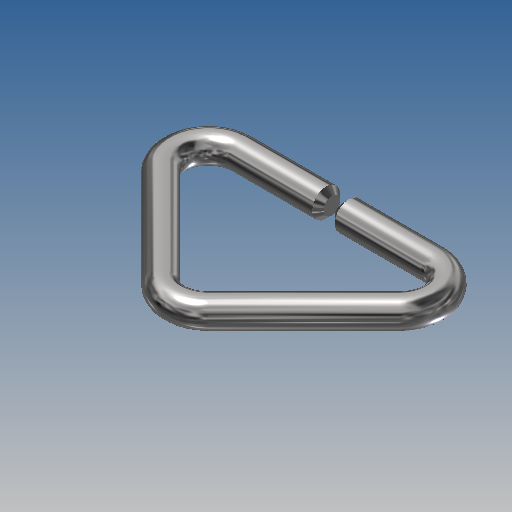
# Autodesk Inventor part: DD_KVD_002_12
Saved by Autodesk Inventor 2017.3 (Build 213256000, 256)
## iProperties
Created: 2023-12-14
Part Number: DD_KVD_002_12
Material: Nerezová ocel
Document SubType Name: Modeling
Designer: Darena
Manufacturer: Standard
Standards Organization: Custom
Density: 8 g/cm^3
Appearance: Pololeštěná
Author: Darena
Autodesk Inventor part; units mm, degrees
ref_plane "YZ Plane" through (0, 0, 0) normal (1, 0, 0) x (0, 1, 0)
ref_plane "XZ Plane" through (0, 0, 0) normal (0, 1, 0) x (-1, 0, 0)
ref_plane "XY Plane" through (0, 0, 0) normal (0, 0, 1) x (1, 0, 0)
sketch "Náčrt2" plane through (0, 0, 0) normal (0, 1, 0) x (-1, 0, 0)
  line L0 (-15, 3.4854) -> (17, 3.4854) construction
  line L1 (17, 3.4854) -> (17, 9.4853) construction
  line L2 (17, 9.4853) -> (-15, 9.4853) construction
  line L3 (20.5, 23.4853) -> (39.8276, 23.4853) construction
  line L4 (20.5, 23.4853) -> (20.5, 35.0341) construction
  line L5 (4.2426, 27.2426) -> (21.2426, 10.2426)
  line L6 (17, 0) -> (-17, 0)
  line L7 (-4.2426, 27.2426) -> (-21.2426, 10.2426)
  line L8 (0, 9.4853) -> (0, 31.4853) construction
  arc A0 (4.2426, 27.2426) -> (-4.2426, 27.2426) centre (0, 23) ccw
  arc A1 (17, 0) -> (21.2426, 10.2426) centre (17, 6) ccw
  arc A2 (-21.2426, 10.2426) -> (-17, 0) centre (-17, 6) ccw
  line L9 (19.1213, 8.1213) -> (2.1213, 25.1213) construction
  arc A3 (2.1213, 25.1213) -> (-2.1213, 25.1213) centre (0, 23) ccw construction
  line L10 (-2.1213, 25.1213) -> (-19.1213, 8.1213) construction
  arc A4 (-19.1213, 8.1213) -> (-17, 3) centre (-17, 6) ccw construction
  line L11 (-17, 3) -> (17, 3) construction
  arc A5 (17, 3) -> (19.1213, 8.1213) centre (17, 6) ccw construction
  line L12 (23.364, 12.364) -> (6.364, 29.364) construction
  arc A6 (6.364, 29.364) -> (-6.364, 29.364) centre (0, 23) ccw construction
  line L13 (-6.364, 29.364) -> (-23.364, 12.364) construction
  arc A7 (-23.364, 12.364) -> (-17, -3) centre (-17, 6) ccw construction
  line L14 (-17, -3) -> (17, -3) construction
  arc A8 (17, -3) -> (23.364, 12.364) centre (17, 6) ccw construction
  circle A9 centre (0, 20.4853) radius 3 construction
  line L15 (0, 9.4853) -> (0, 0) construction
  line L16 (36.2885, 20.7337) -> (33.8584, 23.4853) construction
  line L17 (0, 20.4853) -> (20.2426, 20.4853) construction
  line L18 (-15, 3.4854) -> (-15, 9.4853) construction
  point P0 (0, 0)
  dimension "d5" = 45
  dimension "d6" = 45
  dimension "d7" = 6
  dimension "d8" = 3
  dimension "d9" = 3
  dimension "d10" = 6
  dimension "d12" = 32
  dimension "d13" = 5.9999
  dimension "d23" = 20.5
  dimension "d26" = 34
  dimension "d27" = 14
  dimension "d28" = 3
  constraints: 38 end point, 18 point on circle, 10 centre point, 6 tangent, 5 point on line, 4 horizontal, 3 perpendicular, 2 equal radius, 2 midpoint, 2 vertical, 1 coincident, 1 parallel, 10 other
  measures "d5" angle of L6 L5
  measures "d6" angle of L6 L7
  measures "d7" radius of A0
  measures "d8" distance between parallel lines of L5 L9
  measures "d9" distance between parallel lines of L5 L12
  measures "d10" diameter of A9
  measures "d12" distance of L0.start L0.end
  measures "d13" distance between parallel lines of L2 L0
  measures "d23" distance between parallel lines of L4 L8
  measures "d26" distance of L6.start L6.end
  measures "d27" distance between parallel lines of L3 L2
  measures "d28" distance between parallel lines of L17 L3
sketch "Náčrt3" plane through (0, 0, 0) normal (1, 0, 0) x (0, 1, 0)
  circle A0 centre (0, 0) radius 2.5
  dimension "d14" = 5
  constraints: 1 centre point, 1 coincident
  measures "d14" diameter of A0
sweep "Tažení1" add profiles "Náčrt3" path "Náčrt2"
sketch "Náčrt4" plane through (0, 0, 0) normal (0, 1, 0) x (-1, 0, 0)
  line L0 (17, -2.5) -> (17, 2.5) projected
  line L1 (-17, -2.5) -> (-17, 2.5) projected
  line L2 (-17, 2.5) -> (17, 2.5) projected
  line L3 (-17, -2.5) -> (17, -2.5) projected
  line L4 (-1, 2.5) -> (1, 2.5)
  line L5 (1, 2.5) -> (1, -2.5)
  line L6 (1, -2.5) -> (-1, -2.5)
  line L7 (-1, -2.5) -> (-1, 2.5)
  point P0 (0, 0)
  point P1 (0, 2.5)
  point P2 (0, 2.5)
  point P3 (0, -2.5)
  point P4 (0, -2.5)
  dimension "d17" = 2
  constraints: 8 end point, 4 midpoint, 2 coincident, 2 parallel, 1 horizontal, 1 perpendicular, 1 vertical alignment
  measures "d17" distance between parallel lines of L7 L5
extrude "Vysunutí1" cut sketch "Náčrt4" along normal through all both and the other way through all contours L3 L7 L2 L5
chamfer "Zkosení1" distance 1 angle 45 2 edges at (-1, -2.5, 0) (1, -2.5, 0)
